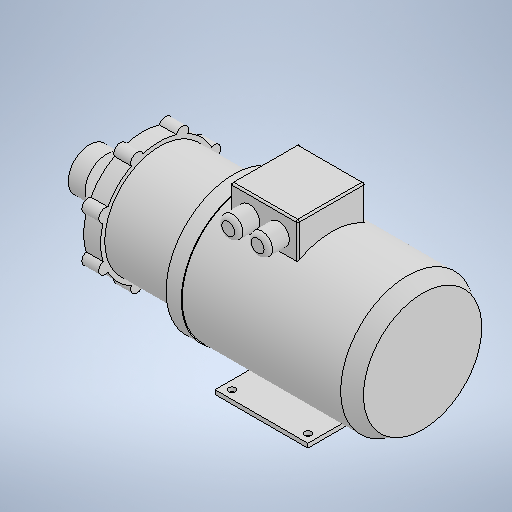
# Autodesk Inventor part: СДР 060 Мотор-редуктор 2.0
Saved by Autodesk Inventor 2025.1 (Build 291241020, 241B)
## iProperties
Created: 2024-04-02
Part Number: СДР 060 Мотор-редуктор 2.0
Material: Типовые
Document SubType Name: Modeling
Designer: pokla
Density: 1 g/cm^3
Appearance: По умолчанию
Author: pokla
Autodesk Inventor part; units mm, degrees
ref_plane "YZ Plane" through (0, 0, 0) normal (1, 0, 0) x (0, 1, 0)
ref_plane "XZ Plane" through (0, 0, 0) normal (0, 1, 0) x (-1, 0, 0)
ref_plane "XY Plane" through (0, 0, 0) normal (0, 0, 1) x (1, 0, 0)
sketch "Эскиз1" plane through (0, 0, 0) normal (0, 1, 0) x (-1, 0, 0)
  line L0 (0, 0) -> (0, -80) construction
  line L1 (0, -80) -> (-9, -80)
  line L2 (-9, -80) -> (-9, -79)
  line L3 (-9, -79) -> (-197, -79)
  line L4 (-197, -79) -> (-215, -70)
  line L5 (-215, -70) -> (-215, 0)
  line L6 (-215, 0) -> (0, 0)
  line L7 (0, -80) -> (9, -80)
  line L8 (9, -80) -> (9, -65)
  line L9 (9, -65) -> (96.6667, -65)
  line L10 (96.6667, -65) -> (96.6667, -70)
  line L11 (116.6667, -70) -> (116.6667, -65)
  line L12 (116.6667, -65) -> (160, -25)
  line L13 (160, -25) -> (180, -25)
  line L14 (180, -25) -> (180, 0)
  line L15 (96.6667, -70) -> (116.6667, -70)
  line L16 (110, -70) -> (110, 0) construction
  line L17 (116.6667, -65) -> (110, -65) construction
  line L18 (103.3333, -65) -> (96.6667, -65) construction
  line L19 (103.3333, -65) -> (110, -65) construction
  line L20 (180, 0) -> (0, 0)
  point P0 (-4.5, -80)
  dimension "d0" = 215
  dimension "d1" = 9
  dimension "d14" = 160
  dimension "d103" = 158
  dimension "d104" = 140
  dimension "d105" = 18
  dimension "d135" = 180
  dimension "d136" = 130
  dimension "d137" = 140
  dimension "d139" = 50
  dimension "d140" = 110
  dimension "d141" = 20
  dimension "d142" = 20
  constraints: 42 end point, 10 perpendicular, 5 collinear, 5 point on line, 2 parallel, 1 horizontal, 1 midpoint, 1 vertical
  measures "d0" distance of L5.end L0.start
  measures "d1" distance of L0.end L1.end
  measures "d14" diameter of point (-4.5, -80) L6
  measures "d103" diameter of L3 L6
  measures "d104" diameter of L4.end L6
  measures "d105" distance from line of L5 L3.end
  measures "d135" distance between parallel lines of L0 L14
  measures "d136" diameter of L9 L6
  measures "d137" diameter of L15 L6
  measures "d139" diameter of L13 L6
  measures "d140" distance from line of L0.end L16
  measures "d141" distance of L12.end L13.end
  measures "d142" distance of L10.end L11.start
revolve "Вращение1" add sketch "Эскиз1" angle 360 about axis through (215, 0, 0) along (-1, 0, 0)
sketch "Эскиз5" plane through (0, 0, 0) normal (0, 1, 0) x (-1, 0, 0)
  line L0 (-197, -79) -> (-197, 79) projected
  line L1 (-9, -79) -> (-9, 79) projected
  line L2 (-27, -40) -> (-107, -40)
  line L3 (-107, -40) -> (-107, 40)
  line L4 (-107, 40) -> (-27, 40)
  line L5 (-27, 40) -> (-27, -40)
  point P0 (0, 0)
  point P1 (-27, 0)
  point P2 (-9, 0)
  dimension "d38" = 80
  dimension "d40" = 18
  constraints: 8 end point, 2 midpoint, 2 parallel, 2 perpendicular, 1 horizontal, 1 horizontal alignment
  measures "d38" distance of L3.end L4.end
  measures "d40" distance between parallel lines of L1 L5
extrude "Выдавливание4" add sketch "Эскиз5" along normal blind 110
sketch "Sketch15" plane through (27, 68.1249, 40) normal (0, 0, 1) x (1, 0, 0)
  circle A0 centre (22.5, 17.8751) radius 12.5
  circle A1 centre (57.5, 17.8751) radius 12.5
  line L0 (80, 41.8751) -> (0, 41.8751) construction
  line L1 (40, 41.8751) -> (40, 0) construction
  line L2 (0, 0) -> (80, 0) construction
  point P0 (-27, -68.1249)
  dimension "d106" = 25
  dimension "d107" = 35
  dimension "d108" = 24
  constraints: 2 centre point, 2 end point, 2 midpoint, 1 equal radius, 1 horizontal alignment, 1 symmetric about line
  measures "d106" diameter of A0
  measures "d107" distance of A1.centre A0.centre
  measures "d108" distance from line of A0.centre L0
extrude "Extrusion14" add sketch "Sketch15" along normal blind 25
fillet "Fillet1" radius 5 2 edges at (37, 86, 65) (72, 86, 65)
fillet "Fillet2" radius 2 8 edges at (27, 89.0624, 40) (67, 110, 40) (107, 89.0624, 40) (107, 110, 0) (67, 110, -40) (27, 110, 0) (107, 89.0624, -40) (27, 89.0624, -40)
sketch "Sketch20" plane through (-116.6667, 0, 0) normal (-1, 0, 0) x (0, 0, 1)
  circle A0 centre (0, 0) radius 70 projected
  circle A1 centre (26.7878, 64.6716) radius 7.5
  line L0 (0, 0) -> (0, 70)
  line L1 (26.7878, 64.6716) -> (0, 0)
  point P0 (19.7149, 67.1664)
  point P1 (33.5532, 61.4344)
  dimension "d143" = 15
  dimension "d144" = 22.5
  constraints: 4 end point, 2 point on circle, 1 centre point, 1 vertical
  measures "d143" diameter of A1
  measures "d144" angle of L0 L1
extrude "Extrusion19" add sketch "Sketch20" against normal up to surface (20 mm away) contours A1 A0
pattern_circular "Circular Pattern1" count 8 over 360 about axis through (-10, 0, 0) along (1, 0, 0) of "Extrusion19"
sketch "Sketch21" plane through (0, 0, 0) normal (0, 1, 0) x (-1, 0, 0)
  line L0 (-145, 66) -> (-35, 66)
  line L1 (-35, 66) -> (-35, -66)
  line L2 (-35, -66) -> (-145, -66)
  line L3 (-145, -66) -> (-145, 66)
  line L4 (-145, 66) -> (-35, -66) construction
  line L5 (-35, 66) -> (-145, -66) construction
  circle A0 centre (-45, -56) radius 4
  line L6 (-35, 0) -> (-145, 0) construction
  line L7 (-90, -66) -> (-90, 66) construction
  circle A1 centre (-45, 56) radius 4
  circle A2 centre (-135, -56) radius 4
  circle A3 centre (-135, 56) radius 4
  point P0 (0, 0)
  point P1 (-90, 0)
  point P2 (-90, 0)
  dimension "d151" = 8
  dimension "d152" = 112
  dimension "d153" = 90
  dimension "d154" = 45
  dimension "d155" = 10
  dimension "d156" = 10
  constraints: 16 end point, 7 midpoint, 4 centre point, 2 horizontal alignment, 2 parallel, 1 equal radius, 1 horizontal, 1 perpendicular, 3 other
  measures "d151" diameter of A0
  measures "d152" distance of A1.centre A0.centre
  measures "d153" distance of A2.centre A0.centre
  measures "d154" horizontal distance of A0.centre point (0, 0)
  measures "d155" distance from line of L1 A0.centre
  measures "d156" distance from line of A0.centre L2
extrude "Extrusion20" add sketch "Sketch21" against normal blind 91
sketch "Sketch22" plane through (35, -91, -66) normal (-1, 0, 0) x (0, 0, 1)
  arc A0 (0, 47.5834) -> (132, 47.5834) centre (66, 91) ccw projected
  line L0 (0, 47.5834) -> (0, 0) projected
  line L1 (132, 0) -> (0, 0) projected
  line L2 (132, 47.5834) -> (132, 0) projected
  line L3 (132, 5) -> (0, 5)
  point P0 (66, 91)
  dimension "d159" = 5
  constraints: 2 end point, 2 point on line, 1 perpendicular
  measures "d159" distance between parallel lines of L1 L3
extrude "Extrusion21" cut sketch "Sketch22" against normal through all contours A0 L2 L3 L0
equation "\"Reductor_angle\" = 180deg"
